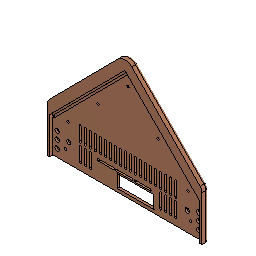
back2_dev (Autodesk Fusion 360 design; units mm, degrees)
Autodesk Fusion 360 part; units mm, degrees
sketch "Skizze1" plane through (0, 0, 0) normal (0, 1, 0) x (1, 0, 0)
  circle A0 centre (0, -97.2038) radius 3.5
  circle A1 centre (47.1436, -49.5962) radius 3.5
  line L0 (118.137, 1.414) -> (116.137, 1.414)
  line L1 (0, -200) -> (0, 115.9522) construction
  line L2 (-116.137, 1.414) -> (-116.137, 3.414)
  line L3 (-118.137, 1.414) -> (-116.137, 1.414)
  circle A2 centre (-98.38, 37) radius 3.5
  circle A3 centre (98.38, 37) radius 3.5
  line L4 (-117.137, 2.414) -> (0, -114.6792) construction
  line L5 (1.065, -116.7355) -> (118.202, 1.3577)
  circle A4 centre (47.1436, -49.5962) radius 1.75
  line L6 (0, -113.5492) -> (116.072, 3.4703)
  line L7 (0, -97.2038) -> (94.2873, -1.9887) construction
  line L8 (-121.38, -20.1074) -> (-10.6584, -131.9185)
  line L9 (-121.38, 55) -> (121.38, 55)
  circle A5 centre (98.38, 37) radius 1.75
  line L10 (116.137, 1.414) -> (118.137, 3.414) construction
  line L11 (-118.137, 3.414) -> (-118.137, 1.414)
  circle A6 centre (-94.2873, -1.9887) radius 1.75
  line L12 (-142.4127, 37) -> (157.273, 37) construction
  line L13 (-114.552, 0) -> (0, -115.6792)
  line L14 (-116.072, 3.4703) -> (0, -113.5492)
  arc A7 (118.202, 1.3577) -> (116.072, 3.4703) centre (117.137, 2.414) ccw
  line L15 (118.137, 3.414) -> (118.137, 1.414)
  line L16 (-94.2873, -1.9887) -> (0, -97.2038) construction
  circle A8 centre (-98.38, 37) radius 1.75
  line L17 (-157.6793, 0) -> (142.763, 0) construction
  arc A9 (-116.072, 3.4703) -> (-118.202, 1.3577) centre (-117.137, 2.414) ccw
  line L18 (106.9019, 1.414) -> (127.3315, 1.414) construction
  line L19 (-118.137, 1.414) -> (-116.137, 3.414) construction
  circle A10 centre (-94.2873, -1.9887) radius 3.5
  line L20 (117.3942, -2.8145) -> (0, -121.364)
  line L21 (117.3942, -2.8145) -> (121.38, -2.8145)
  line L22 (-121.38, -20.1074) -> (-121.38, 55)
  line L23 (0, -115.6792) -> (114.552, 0)
  line L24 (-118.137, -2.8145) -> (-118.137, 55)
  line L25 (-118.202, 1.3577) -> (-1.065, -116.7355)
  line L26 (-114.552, 0) -> (-117.3942, -2.8145)
  line L27 (0, -121.364) -> (-117.3942, -2.8145)
  line L28 (118.137, -2.8145) -> (118.137, 55)
  circle A11 centre (94.2873, -1.9887) radius 3.5
  line L29 (121.38, -20.1074) -> (121.38, 55)
  line L30 (-117.3942, -2.8145) -> (-121.38, -2.8145)
  line L31 (-126.7315, 1.414) -> (-100.8539, 1.414) construction
  line L32 (114.552, 0) -> (117.3942, -2.8145)
  line L33 (-118.137, 3.414) -> (-116.137, 1.414) construction
  line L34 (116.137, 1.414) -> (116.137, 3.414)
  circle A12 centre (94.2873, -1.9887) radius 1.75
  line L35 (116.137, 3.414) -> (118.137, 3.414)
  line L36 (-116.137, 3.414) -> (-118.137, 3.414)
  line L37 (116.137, 3.414) -> (118.137, 1.414) construction
  line L38 (10.6584, -131.9185) -> (121.38, -20.1074)
  circle A13 centre (-47.1436, -49.5962) radius 1.75
  line L39 (117.137, 2.414) -> (0, -114.6792) construction
  circle A14 centre (-47.1436, -49.5962) radius 3.5
  arc A15 (-10.6584, -131.9185) -> (10.6584, -131.9185) centre (0, -121.364) ccw
  circle A16 centre (0, -97.2038) radius 1.75
  line L40 (111.38, -50) -> (111.38, 95) construction
  line L41 (-111.38, -45.2078) -> (-111.38, 108.225) construction
  circle A17 centre (111.38, 43) radius 3.5
  circle A18 centre (111.38, 31) radius 3.5
  circle A19 centre (111.38, 19) radius 3.5
  circle A20 centre (-111.38, 43) radius 3.5
  circle A21 centre (-111.38, 31) radius 3.5
  circle A22 centre (-111.38, 19) radius 3.5
  circle A23 centre (93.137, 25) radius 3.5
  circle A24 centre (-93.137, 25) radius 3.5
  line L42 (40.8, 29.9) -> (-16.8, 29.9)
  line L43 (-16.8, 29.9) -> (-16.8, 50)
  line L44 (-16.8, 50) -> (40.8, 50)
  line L45 (40.8, 50) -> (40.8, 29.9)
  line L46 (95.5507, 5) -> (-73.9342, 5) construction
  line L47 (73.5, 16) -> (76.5, 16) construction
  line L48 (76.5, 16) -> (76.5, -6)
  line L49 (76.5, -6) -> (73.5, -6) construction
  line L50 (73.5, -6) -> (73.5, 16)
  line L51 (73.5, 16) -> (76.5, -6) construction
  line L52 (76.5, 16) -> (73.5, -6) construction
  arc A25 (76.5, 16) -> (73.5, 16) centre (75, 16) ccw
  arc A26 (73.5, -6) -> (76.5, -6) centre (75, -6) ccw
  line L53 (65.6053, -6) -> (65.6053, 16)
  arc A27 (65.6053, -6) -> (68.6053, -6) centre (67.1053, -6) ccw
  line L54 (68.6053, 16) -> (68.6053, -6)
  arc A28 (68.6053, 16) -> (65.6053, 16) centre (67.1053, 16) ccw
  line L55 (57.7105, -6) -> (57.7105, 16)
  arc A29 (57.7105, -6) -> (60.7105, -6) centre (59.2105, -6) ccw
  line L56 (60.7105, 16) -> (60.7105, -6)
  arc A30 (60.7105, 16) -> (57.7105, 16) centre (59.2105, 16) ccw
  line L57 (49.8158, -6) -> (49.8158, 16)
  arc A31 (49.8158, -6) -> (52.8158, -6) centre (51.3158, -6) ccw
  line L58 (52.8158, 16) -> (52.8158, -6)
  arc A32 (52.8158, 16) -> (49.8158, 16) centre (51.3158, 16) ccw
  line L59 (41.9211, -6) -> (41.9211, 16)
  arc A33 (41.9211, -6) -> (44.9211, -6) centre (43.4211, -6) ccw
  line L60 (44.9211, 16) -> (44.9211, -6)
  arc A34 (44.9211, 16) -> (41.9211, 16) centre (43.4211, 16) ccw
  line L61 (34.0263, -6) -> (34.0263, 16)
  arc A35 (34.0263, -6) -> (37.0263, -6) centre (35.5263, -6) ccw
  line L62 (37.0263, 16) -> (37.0263, -6)
  arc A36 (37.0263, 16) -> (34.0263, 16) centre (35.5263, 16) ccw
  line L63 (26.1316, -6) -> (26.1316, 16)
  arc A37 (26.1316, -6) -> (29.1316, -6) centre (27.6316, -6) ccw
  line L64 (29.1316, 16) -> (29.1316, -6)
  arc A38 (29.1316, 16) -> (26.1316, 16) centre (27.6316, 16) ccw
  line L65 (18.2368, -6) -> (18.2368, 16)
  arc A39 (18.2368, -6) -> (21.2368, -6) centre (19.7368, -6) ccw
  line L66 (21.2368, 16) -> (21.2368, -6)
  arc A40 (21.2368, 16) -> (18.2368, 16) centre (19.7368, 16) ccw
  line L67 (10.3421, -6) -> (10.3421, 16)
  arc A41 (10.3421, -6) -> (13.3421, -6) centre (11.8421, -6) ccw
  line L68 (13.3421, 16) -> (13.3421, -6)
  arc A42 (13.3421, 16) -> (10.3421, 16) centre (11.8421, 16) ccw
  line L69 (2.4474, -6) -> (2.4474, 16)
  arc A43 (2.4474, -6) -> (5.4474, -6) centre (3.9474, -6) ccw
  line L70 (5.4474, 16) -> (5.4474, -6)
  arc A44 (5.4474, 16) -> (2.4474, 16) centre (3.9474, 16) ccw
  line L71 (-5.4474, -6) -> (-5.4474, 16)
  arc A45 (-5.4474, -6) -> (-2.4474, -6) centre (-3.9474, -6) ccw
  line L72 (-2.4474, 16) -> (-2.4474, -6)
  arc A46 (-2.4474, 16) -> (-5.4474, 16) centre (-3.9474, 16) ccw
  line L73 (-13.3421, -6) -> (-13.3421, 16)
  arc A47 (-13.3421, -6) -> (-10.3421, -6) centre (-11.8421, -6) ccw
  line L74 (-10.3421, 16) -> (-10.3421, -6)
  arc A48 (-10.3421, 16) -> (-13.3421, 16) centre (-11.8421, 16) ccw
  line L75 (-21.2368, -6) -> (-21.2368, 16)
  arc A49 (-21.2368, -6) -> (-18.2368, -6) centre (-19.7368, -6) ccw
  line L76 (-18.2368, 16) -> (-18.2368, -6)
  arc A50 (-18.2368, 16) -> (-21.2368, 16) centre (-19.7368, 16) ccw
  line L77 (-29.1316, -6) -> (-29.1316, 16)
  arc A51 (-29.1316, -6) -> (-26.1316, -6) centre (-27.6316, -6) ccw
  line L78 (-26.1316, 16) -> (-26.1316, -6)
  arc A52 (-26.1316, 16) -> (-29.1316, 16) centre (-27.6316, 16) ccw
  line L79 (-37.0263, -6) -> (-37.0263, 16)
  arc A53 (-37.0263, -6) -> (-34.0263, -6) centre (-35.5263, -6) ccw
  line L80 (-34.0263, 16) -> (-34.0263, -6)
  arc A54 (-34.0263, 16) -> (-37.0263, 16) centre (-35.5263, 16) ccw
  line L81 (-44.9211, -6) -> (-44.9211, 16)
  arc A55 (-44.9211, -6) -> (-41.9211, -6) centre (-43.4211, -6) ccw
  line L82 (-41.9211, 16) -> (-41.9211, -6)
  arc A56 (-41.9211, 16) -> (-44.9211, 16) centre (-43.4211, 16) ccw
  line L83 (-52.8158, -6) -> (-52.8158, 16)
  arc A57 (-52.8158, -6) -> (-49.8158, -6) centre (-51.3158, -6) ccw
  line L84 (-49.8158, 16) -> (-49.8158, -6)
  arc A58 (-49.8158, 16) -> (-52.8158, 16) centre (-51.3158, 16) ccw
  line L85 (-60.7105, -6) -> (-60.7105, 16)
  arc A59 (-60.7105, -6) -> (-57.7105, -6) centre (-59.2105, -6) ccw
  line L86 (-57.7105, 16) -> (-57.7105, -6)
  arc A60 (-57.7105, 16) -> (-60.7105, 16) centre (-59.2105, 16) ccw
  line L87 (-68.6053, -6) -> (-68.6053, 16)
  arc A61 (-68.6053, -6) -> (-65.6053, -6) centre (-67.1053, -6) ccw
  line L88 (-65.6053, 16) -> (-65.6053, -6)
  arc A62 (-65.6053, 16) -> (-68.6053, 16) centre (-67.1053, 16) ccw
  line L89 (-76.5, -6) -> (-76.5, 16)
  arc A63 (-76.5, -6) -> (-73.5, -6) centre (-75, -6) ccw
  line L90 (-73.5, 16) -> (-73.5, -6)
  arc A64 (-73.5, 16) -> (-76.5, 16) centre (-75, 16) ccw
  line L91 (86, 33) -> (-83.4948, 33) construction
  line L92 (73.5, 44) -> (76.5, 44) construction
  line L93 (76.5, 44) -> (76.5, 22)
  line L94 (76.5, 22) -> (73.5, 22) construction
  line L95 (73.5, 22) -> (73.5, 44)
  line L96 (73.5, 44) -> (76.5, 22) construction
  line L97 (76.5, 44) -> (73.5, 22) construction
  arc A65 (73.5, 22) -> (76.5, 22) centre (75, 22) ccw
  arc A66 (76.5, 44) -> (73.5, 44) centre (75, 44) ccw
  line L98 (65.605, 22) -> (65.605, 44)
  arc A67 (65.605, 22) -> (68.605, 22) centre (67.105, 22) ccw
  line L99 (68.605, 44) -> (68.605, 22)
  arc A68 (68.605, 44) -> (65.605, 44) centre (67.105, 44) ccw
  line L100 (57.71, 22) -> (57.71, 44)
  arc A69 (57.71, 22) -> (60.71, 22) centre (59.21, 22) ccw
  line L101 (60.71, 44) -> (60.71, 22)
  arc A70 (60.71, 44) -> (57.71, 44) centre (59.21, 44) ccw
  line L102 (49.815, 22) -> (49.815, 44)
  arc A71 (49.815, 22) -> (52.815, 22) centre (51.315, 22) ccw
  line L103 (52.815, 44) -> (52.815, 22)
  arc A72 (52.815, 44) -> (49.815, 44) centre (51.315, 44) ccw
  line L104 (-76.5, 44) -> (-73.5, 44) construction
  line L105 (-73.5, 44) -> (-73.5, 22)
  line L106 (-73.5, 22) -> (-76.5, 22) construction
  line L107 (-76.5, 22) -> (-76.5, 44)
  line L108 (-76.5, 44) -> (-73.5, 22) construction
  line L109 (-73.5, 44) -> (-76.5, 22) construction
  arc A73 (-76.5, 22) -> (-73.5, 22) centre (-75, 22) ccw
  arc A74 (-73.5, 44) -> (-76.5, 44) centre (-75, 44) ccw
  line L110 (-68.605, 22) -> (-68.605, 44)
  arc A75 (-68.605, 22) -> (-65.605, 22) centre (-67.105, 22) ccw
  line L111 (-65.605, 44) -> (-65.605, 22)
  arc A76 (-65.605, 44) -> (-68.605, 44) centre (-67.105, 44) ccw
  line L112 (-60.71, 22) -> (-60.71, 44)
  arc A77 (-60.71, 22) -> (-57.71, 22) centre (-59.21, 22) ccw
  line L113 (-57.71, 44) -> (-57.71, 22)
  arc A78 (-57.71, 44) -> (-60.71, 44) centre (-59.21, 44) ccw
  line L114 (46.3033, 26.1) -> (-55, 26.1) construction
  line L115 (-18, 27.6) -> (6, 27.6)
  line L116 (6, 27.6) -> (6, 24.6) construction
  line L117 (6, 24.6) -> (-18, 24.6)
  line L118 (-18, 24.6) -> (-18, 27.6) construction
  line L119 (-18, 27.6) -> (6, 24.6) construction
  line L120 (6, 27.6) -> (-18, 24.6) construction
  arc A79 (6, 24.6) -> (6, 27.6) centre (6, 26.1) ccw
  arc A80 (-17.6308, 27.5538) -> (-18, 24.6) centre (-18, 26.1) ccw
  line L121 (-47, 27.6) -> (-23, 27.6)
  line L122 (-23, 27.6) -> (-23, 24.6) construction
  line L123 (-23, 24.6) -> (-47, 24.6)
  line L124 (-47, 24.6) -> (-47, 27.6) construction
  line L125 (-47, 27.6) -> (-23, 24.6) construction
  line L126 (-23, 27.6) -> (-47, 24.6) construction
  line L127 (11, 27.6) -> (35, 27.6)
  line L128 (35, 27.6) -> (35, 24.6) construction
  line L129 (35, 24.6) -> (11, 24.6)
  line L130 (11, 24.6) -> (11, 27.6) construction
  line L131 (11, 27.6) -> (35, 24.6) construction
  line L132 (35, 27.6) -> (11, 24.6) construction
  arc A81 (-47, 27.6) -> (-47, 24.6) centre (-47, 26.1) ccw
  arc A82 (-23, 24.6) -> (-23, 27.6) centre (-23, 26.1) ccw
  arc A83 (11, 27.6) -> (11, 24.6) centre (11, 26.1) ccw
  arc A84 (35, 24.6) -> (35, 27.6) centre (35, 26.1) ccw
  circle A85 centre (0, -115.6792) radius 1
  circle A86 centre (0, -115.6792) radius 1.5 construction
  arc A87 (-1.065, -116.7355) -> (1.065, -116.7355) centre (0, -115.6792) ccw
  point P0 (0, -97.2038)
  point P1 (114.552, 0)
  point P2 (-114.552, 0)
  point P3 (-117.137, 2.414)
  point P4 (117.137, 2.414)
  point P5 (75, 5)
  point P6 (75, 33)
  point P7 (-75, 33)
  point P8 (-6, 26.1)
  point P9 (-35, 26.1)
  point P10 (23, 26.1)
  point P11 (-6, 26.1)
  dimension "d1" = 55
  dimension "d2" = 121.38
  dimension "d3" = 121.38
  dimension "d4" = 3.243
  dimension "d5" = 3.243
  dimension "d6" = 1.414
  dimension "d7" = 1.414
  dimension "d8" = 2
  dimension "d9" = 2
  dimension "d10" = 2
  dimension "d11" = 2
  dimension "d12" = 6.828
  dimension "d13" = 6.828
  dimension "d15" = 4
  dimension "d16" = 4
  dimension "d17" = 15
  dimension "d18" = 15
  dimension "d19" = 15
  dimension "d20" = 13
  dimension "d21" = 13
  dimension "d22" = 3.5
  dimension "d23" = 7
  dimension "d24" = 3.5
  dimension "d25" = 3.5
  dimension "d26" = 67
  dimension "d28" = 3.5
  dimension "d29" = 3.5
  dimension "d30" = 67
  dimension "d32" = 7
  dimension "d33" = 7
  dimension "d34" = 7
  dimension "d35" = 7
  dimension "d36" = 18
  dimension "d37" = 23
  dimension "d38" = 23
  dimension "d39" = 3.5
  dimension "d40" = 7
  dimension "d41" = 3.5
  dimension "d42" = 7
  dimension "d44" = 1.5
  dimension "d46" = 1.5
  dimension "d47" = 10
  dimension "d48" = 10
  dimension "d49" = 7
  dimension "d50" = 7
  dimension "d51" = 7
  dimension "d52" = 12
  dimension "d53" = 12
  dimension "d54" = 12
  dimension "d55" = 7
  dimension "d56" = 7
  dimension "d57" = 7
  dimension "d58" = 12
  dimension "d59" = 12
  dimension "d60" = 12
  dimension "d61" = 7
  dimension "d62" = 28.243
  dimension "d63" = 30
  dimension "d64" = 28.243
  dimension "d65" = 30
  dimension "d66" = 7
  dimension "d67" = 5
  dimension "d68" = 20.1
  dimension "d69" = 40.8
  dimension "d70" = 16.8
  dimension "d87" = 50
  dimension "d88" = 75
  dimension "d89" = 3
  dimension "d90" = 22
  dimension "d93" = -150
  dimension "d94" = 0
  dimension "d95" = 22
  dimension "d96" = 3
  dimension "d97" = 75
  dimension "d98" = 22
  dimension "d101" = -23.685
  dimension "d102" = 0
  dimension "d103" = 3
  dimension "d104" = 22
  dimension "d105" = 75
  dimension "d108" = 15.79
  dimension "d109" = 0
  dimension "d110" = 28.9
  dimension "d111" = 3
  dimension "d112" = 24
  dimension "d113" = 3
  dimension "d114" = 3
  dimension "d115" = 24
  dimension "d116" = 24
  dimension "d117" = 29
  dimension "d118" = 29
  dimension "d120" = 6
  dimension "d121" = 162.8
  dimension "d122" = 2
  dimension "d123" = 3
  dimension "d125" = 67
  dimension "d126" = 67
  constraint horizontal L17
  constraint perpendicular L1 L17
  constraint coincident origin L1
  constraint coincident origin L17
  constraint horizontal L9
  constraint perpendicular L17 L22
  constraint perpendicular L9 L29
  constraint coincident L9.end L29.end
  constraint coincident L9.start L22.end
  constraint coincident L24.end L9
  constraint perpendicular L9 L24
  constraint coincident L28.end L9
  constraint perpendicular L9 L28
  constraint perpendicular L24 L31
  constraint perpendicular L18 L29
  constraint horizontal L3
  constraint vertical L2
  constraint horizontal L36
  constraint vertical L11
  constraint coincident L3.start L31
  constraint coincident L3.start L24
  constraint horizontal L0
  constraint vertical L34
  constraint horizontal L35
  constraint vertical L15
  constraint coincident L0.start L18
  constraint coincident L0.start L28
  constraint coincident P2 L17
  constraint coincident P1 L17
  constraint coincident P2 L13.start
  constraint coincident L13.end L1
  constraint coincident P1 L23.end
  constraint perpendicular L13 L26
  constraint coincident L30.end L22
  constraint perpendicular L22 L30
  constraint perpendicular L23 L32
  constraint coincident L21.end L29
  constraint perpendicular L21 L29
  constraint coincident L24.start L30
  constraint coincident L28.start L21
  constraint coincident L20.end L1
  constraint parallel L13 L27
  constraint coincident L8.start L22
  constraint coincident L38.end L29
  constraint parallel L20 L38
  constraint parallel L8 L27
  constraint coincident L8.start L22.start
  constraint coincident L29.start L38.end
  constraint tangent L8 A15
  constraint tangent L38 A15
  constraint parallel L13 L16
  constraint parallel L7 L23
  constraint coincident P0 L7
  constraint coincident P0 L16
  constraint coincident P0 A0.centre
  constraint concentric A0 A16
  constraint coincident A1.centre L7
  constraint coincident A11.centre L7
  constraint coincident A13.centre L16
  constraint coincident A6.centre L16
  constraint concentric A6 A10
  constraint concentric A13 A14
  constraint concentric A1 A4
  constraint concentric A11 A12
  constraint perpendicular L12 L22
  constraint coincident A3.centre L12
  constraint concentric A3 A5
  constraint coincident A2.centre L12
  constraint concentric A2 A8
  constraint coincident L15.start L10
  constraint coincident L0.end L10
  constraint coincident L34.end L37
  constraint coincident L0.start L37
  constraint coincident L10.start L0
  constraint coincident L34.end L35
  constraint coincident L10.end L35
  constraint midpoint P4 L10
  constraint coincident P4 A7.centre
  constraint midpoint P3 L33
  constraint coincident P3 L4.start
  constraint tangent L5 A7
  constraint coincident L5.end A7.start
  constraint tangent A9 L25
  constraint coincident A9.end L25.start
  constraint coincident L6.start L1
  constraint tangent L6 A7
  constraint coincident L6.end A7.end
  constraint parallel L5 L6
  constraint tangent L14 A9
  constraint coincident L14.start A9.start
  constraint perpendicular L9 L40
  constraint perpendicular L9 L41
  constraint coincident L40 A17.centre
  constraint coincident L40 A18.centre
  constraint coincident L40 A19.centre
  constraint coincident L41 A20.centre
  constraint coincident L41 A21.centre
  constraint coincident L41 A22.centre
  constraint horizontal L42
  constraint vertical L43
  constraint horizontal L44
  constraint vertical L45
  constraint parallel L9 L46
  constraint horizontal L47
  constraint perpendicular L47 L48
  constraint parallel L47 L49
  constraint parallel L48 L50
  constraint coincident L51 P5
  constraint coincident L52 P5
  constraint coincident L46 P5
  constraint coincident L47 A25.centre
  constraint coincident L49 A26.centre
  constraint horizontal L49.end L50.start
  constraint coincident L50 L49.end
  constraint coincident L50 L47.start
  constraint coincident L47.start L50.end
  constraint parallel L12 L91
  constraint horizontal L92
  constraint perpendicular L92 L93
  constraint parallel L92 L94
  constraint parallel L93 L95
  constraint coincident L96 P6
  constraint coincident L97 P6
  constraint coincident L91 P6
  constraint coincident L94 A65.centre
  constraint coincident L92 A66.centre
  constraint coincident L92.start L95.end
  constraint coincident L94.end L95.start
  constraint horizontal L104
  constraint perpendicular L104 L105
  constraint parallel L104 L106
  constraint parallel L105 L107
  constraint coincident L108 P7
  constraint coincident L109 P7
  constraint coincident L91 P7
  constraint coincident L106 A73.centre
  constraint coincident L104 A74.centre
  constraint coincident L104.end L105.start
  constraint coincident L105.end L106.start
  constraint horizontal L114
  constraint horizontal L115
  constraint perpendicular L115 L116
  constraint parallel L115 L117
  constraint parallel L116 L118
  constraint midpoint L116 A79.centre
  constraint coincident L119 A80.start
  constraint midpoint L118 A80.centre
  constraint horizontal L121
  constraint perpendicular L121 L122
  constraint parallel L121 L123
  constraint parallel L122 L124
  constraint coincident L125 P9
  constraint coincident L126 P9
  constraint coincident L114 P9
  constraint horizontal L127
  constraint perpendicular L127 L128
  constraint parallel L127 L129
  constraint parallel L128 L130
  constraint coincident L131 P10
  constraint coincident L132 P10
  constraint coincident L114 P10
  constraint midpoint L124 A81.centre
  constraint midpoint L122 A82.centre
  constraint midpoint L130 A83.centre
  constraint midpoint L128 A84.centre
  constraint midpoint L120 P11
  constraint coincident P11 P8
  constraint coincident L114 P11
  constraint coincident L13.end L23.start
  constraint concentric A85 A86
  constraint tangent L5 A86
  constraint coincident L5.start A86
  constraint tangent L25 A86
  constraint coincident L25.end A86
  constraint coincident A6.centre L16.start
  constraint coincident L7.end A11.centre
  measures "d1" distance of L9 L17
  measures "d2" distance of L1 L22
  measures "d3" distance of L1 L29
  measures "d4" distance of L28 L29
  measures "d5" distance of L22 L24
  measures "d6" distance of L17 L31
  measures "d7" distance of L17 L18
  measures "d8" distance of L28 L34
  measures "d9" distance of L0 L35
  measures "d10" distance of L3 L36
  measures "d11" distance of L2 L11
  measures "d12" distance of P2 L22
  measures "d13" distance of P1 L29
  measures "d15" distance of L26.end P2
  measures "d16" distance of P1 L20.start
  measures "d17" distance of L20 L38
  measures "d18" radius of A15
  measures "d19" distance of L8 L27
  measures "d20" distance of L7 L23
  measures "d21" distance of L13 L16
  measures "d22" diameter of A16
  measures "d23" diameter of A0
  measures "d24" diameter of A12
  measures "d25" diameter of A4
  measures "d26" distance of A1.centre L7.end
  measures "d28" diameter of A6
  measures "d29" diameter of A13
  measures "d30" distance of A13.centre A6.centre
  measures "d32" diameter of A11
  measures "d33" diameter of A1
  measures "d34" diameter of A14
  measures "d35" diameter of A10
  measures "d36" distance of L9 L12
  measures "d37" distance of A2.centre L22
  measures "d38" distance of A3.centre L29
  measures "d39" diameter of A5
  measures "d40" diameter of A3
  measures "d41" diameter of A8
  measures "d42" diameter of A2
  measures "d44" radius of A7
  measures "d46" radius of A9
  measures "d47" distance of L22 L41
  measures "d48" distance of L29 L40
  measures "d49" diameter of A20
  measures "d50" diameter of A21
  measures "d51" diameter of A22
  measures "d52" distance of L9 A20.centre
  measures "d53" distance of A20.centre A21.centre
  measures "d54" distance of A21.centre A22.centre
  measures "d55" diameter of A19
  measures "d56" diameter of A18
  measures "d57" diameter of A17
  measures "d58" distance of L9 A17.centre
  measures "d59" distance of A17.centre A18.centre
  measures "d60" distance of A18.centre A19.centre
  measures "d61" diameter of A24
  measures "d62" distance of L22 A24.centre
  measures "d63" distance of L9 A24.centre
  measures "d64" distance of L29 A23.centre
  measures "d65" distance of L9 A23.centre
  measures "d66" diameter of A23
  measures "d67" distance of L9 L44
  measures "d68" distance of L42 L44
  measures "d69" distance of L1 L45
  measures "d70" distance of L1 L43
  measures "d87" distance of L9 L46
  measures "d88" distance of L1 P5
  measures "d89" distance of L48 L50
  measures "d90" distance of L47 L49
  measures "d95" distance of L9 L91
  measures "d96" distance of L93 L95
  measures "d97" distance of L1 P6
  measures "d98" distance of L92 L94
  measures "d103" distance of L105 L107
  measures "d104" distance of L104 L106
  measures "d105" distance of L1 P7
  measures "d110" distance of L9 L114
  measures "d111" distance of L115 L117
  measures "d112" distance of L116 L118
  measures "d113" distance of L127 L129
  measures "d114" distance of L121 L123
  measures "d115" distance of L122 L124
  measures "d116" distance of L128 L130
  measures "d117" distance of P11 P10
  measures "d118" distance of P11 P9
  measures "d120" distance of L1 P11
  measures "d121" distance of L13.end L32
  measures "d122" diameter of A85
  measures "d123" diameter of A86
  measures "d125" distance of P0 A1.centre
  measures "d126" distance of P0 A13.centre
extrude "Extrusion1" add sketch "Skizze1" along normal blind 5 contours L0 L2 L3 L5 L6 L13 L14 A7 A9 L23 L24 L25 L26 L28 L32 L34 L35 L36 A85 | L0 L15 L28 L34 L35 | L5 A7 L15 L28 | L5 L21 L28 L32 | L5 L9 A7 L21 L28 L29 | L6 L9 L14 A7 A9 L24 L28 | L5 L20 L25 L26 L27 L32 A87 | L5 L13 L23 L25 L26 L32 A85 A87 | L8 L20 L21 L22 L27 L29 L30 L38 A15 | L9 A9 L22 L24 L25 L30 | L13 L23 A85 | L13 L23 A85 | L11 A9 L24 L25 | L24 L25 L26 L30 | L2 L3 L11 L24 L36 | A17 | A18 | A19 | A20 | A21 | A22 | A23 | A24
chamfer "Fase1" distance 1 angle 45 4 edges at (12, 5, -50) (40.8, 5, -39.95) (12, 5, -29.9) (-16.8, 5, -39.95)
extrude "Extrusion2" add sketch "Skizze1" along normal blind 3 contours A0 | A1 | A2 | A3 | A10 | A11 | A14
extrude "Extrusion3" add sketch "Skizze1" against normal blind 5 contours L5 A7 L15 L28 | L5 L9 A7 L21 L28 L29 | L8 L20 L21 L22 L27 L29 L30 L38 A15 | L9 A9 L22 L24 L25 L30 | L11 A9 L24 L25
extrude "Extrusion4" cut sketch "Skizze1" along normal blind 2 contours L0 L2 L3 L5 L6 L13 L14 A7 A9 L23 L24 L25 L26 L28 L32 L34 L35 L36 A85 | L0 L15 L28 L34 L35 | L5 L13 L23 L25 L26 L32 A85 A87 | L13 L23 A85 | L13 L23 A85 | L2 L3 L11 L24 L36
extrude "Extrusion5" cut sketch "Skizze1" along normal blind 3 contours A17 | A18 | A19 | A20 | A21 | A22 | A23 | A24
fillet "Abrundung1" radius 10 2 edges at (121.38, 0, 20.1074) (-121.38, 0, 20.1074)
fillet "Abrundung2" radius 4 7 edges at (-121.38, 5, -19.503) (-120.6281, 5, 19.7981) (-64.572, 5, 77.4744) (0, 5, 136.364) (64.572, 5, 77.4744) (120.6281, 5, 19.7981) (121.38, 5, -19.503)
move_face "Flächen versetzen1" offset -0.2 2 faces at (-39.1314, -1.6667, 81.8475) (78.2628, -3.3333, 42.331)
equation "d101 = ( -7.895 * 3 ) * 1 mm"
equation "d108 = ( 2 * 7.895 ) * 1 mm"
named bodies: "back2_dev"
